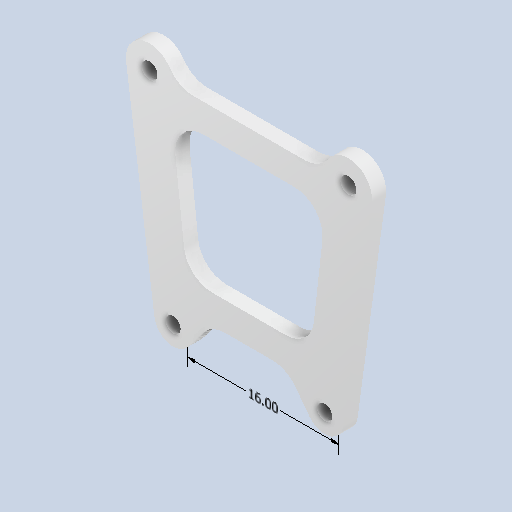
# Autodesk Inventor part: elbow
Saved by Autodesk Inventor 2024.1 (Build 281209000, 209)
## iProperties
Created: 2024-02-14
Part Number: elbow
Material: アルミニウム 6061
Document SubType Name: Modeling
Designer: hibik
Density: 2.7 g/cm^3
Appearance: アルミニウム - フラット
Author: hibik
Autodesk Inventor part; units mm, degrees
ref_plane "YZ Plane" through (0, 0, 0) normal (1, 0, 0) x (0, 1, 0)
ref_plane "XZ Plane" through (0, 0, 0) normal (0, 1, 0) x (-1, 0, 0)
ref_plane "XY Plane" through (0, 0, 0) normal (0, 0, 1) x (1, 0, 0)
sketch "スケッチ2" plane through (0, 0, 0) normal (0, 0, 1) x (1, 0, 0)
  line L0 (0, 0) -> (26, 0)
  line L1 (26, 0) -> (26, 33)
  line L2 (26, 33) -> (0, 33)
  line L3 (0, 33) -> (0, 0)
  line L4 (0, 0) -> (26, 0)
  line L5 (26, 0) -> (26, 24)
  line L6 (26, 24) -> (0, 24) construction
  line L7 (0, 24) -> (0, 0)
  circle A0 centre (13, 24) radius 13
  circle A1 centre (13, 24) radius 6.25
  line L8 (26, 0) -> (0, 0)
  line L9 (26, 24.5219) -> (26, -21)
  line L10 (26, -21) -> (0, -21)
  line L11 (0, -21) -> (0, 24)
  circle A2 centre (5, -19) radius 0.8
  circle A3 centre (21, -19) radius 0.8
  line L12 (0, 24) -> (26, 24)
  point P0 (22.3808, 33)
  point P1 (3.6192, 33)
  point P2 (0, 0)
  point P3 (26, 24)
  point P4 (0, 24)
  point P5 (6.75, 24)
  point P6 (19, 22.25)
  point P7 (19.25, 24)
  dimension "d0" = 26
  dimension "d1" = 33
  dimension "d2" = 24
  dimension "d3" = 12.5
  dimension "d14" = 26
  dimension "d17" = 1.6
  dimension "d18" = 1.6
  dimension "d19" = 2
  dimension "d20" = 2
  dimension "d21" = 5
  dimension "d22" = 5
  dimension "d23" = 13
  dimension "d25" = 45
  dimension "d26" = 0
  constraints: 26 end point, 5 parallel, 3 centre point, 3 horizontal, 3 perpendicular, 2 midpoint, 2 point on line, 1 coincident, 3 other
  measures "d0" distance of L1.end L2.end
  measures "d1" distance of L2.end L0.start
  measures "d2" distance between parallel lines of L0 L6
  measures "d3" diameter of A1
  measures "d14" distance between parallel lines of L11 L9
  measures "d17" diameter of A2
  measures "d18" diameter of A3
  measures "d19" distance from line of A2.centre L10
  measures "d20" distance from line of L10 A3.centre
  measures "d21" distance from line of L11 A2.centre
  measures "d22" distance from line of L9 A3.centre
  measures "d23" distance from line of L11 A1.centre
  measures "d25" distance between parallel lines of L10 L12
  measures "d26" distance between parallel lines of L9 L1
extrude "押し出し1" add sketch "スケッチ2" along normal blind 1.5 contours L3 A0 L1 L0 | L0 L9 L10 L11 | L12 A1 A0 | A0 L2 L12 A1 | A0 L2 L1 | L12 A1 | A1 L12
sketch "スケッチ3" plane through (0, 0, 0) normal (0, 0, -1) x (-1, 0, 0)
  circle A0 centre (-2.5, 24) radius 0.85 projected
  circle A1 centre (-23.5, 24) radius 0.85 projected
  circle A2 centre (-23.5, 3) radius 0.85 projected
  circle A3 centre (-2.5, 3) radius 0.85 projected
  circle A4 centre (-13, 24) radius 6.25 projected
  line L0 (-2.5, 24) -> (-23.5, 24)
  line L1 (-23.5, 24) -> (-23.5, 3)
  line L2 (-23.5, 3) -> (-2.5, 3)
  line L3 (-2.5, 3) -> (-2.5, 24)
  circle A5 centre (-13, 24) radius 10.25
  line L4 (-5.5, 24) -> (-20.5, 24)
  line L5 (-20.5, 24) -> (-20.5, 3)
  line L6 (-20.5, 3) -> (-5.5, 3)
  line L7 (-5.5, 3) -> (-5.5, 24)
  arc A6 (0, 24) -> (-3.6192, 33) centre (-13, 24) ccw projected
  line L8 (-26, 33) -> (-3.6192, 33) projected
  line L9 (-26, -21) -> (-26, 33) projected
  line L10 (0, -21) -> (-26, -21) projected
  line L11 (0, 24) -> (0, -21) projected
  circle A7 centre (-5, -19) radius 0.8 projected
  circle A8 centre (-21, -19) radius 0.8 projected
  line L12 (-37.149, 0) -> (-22.2321, 0)
  line L13 (-22.2321, 0) -> (-8, 0)
  circle A9 centre (-23.5, 3) radius 2.5
  circle A10 centre (-2.5, 3) radius 2.5
  line L14 (-21.5265, 4.5347) -> (-18, 0)
  line L15 (-4.4735, 4.5347) -> (-8, 0)
  line L16 (-18, 0) -> (-8, 0)
  circle A11 centre (-21, -19) radius 2
  circle A12 centre (-5, -19) radius 2
  line L17 (-26, -21) -> (-26, 33) projected
  line L18 (-19.4, -20.2) -> (-17, -17)
  line L19 (-17, -17) -> (-9, -17)
  line L20 (-9, -17) -> (-6.6, -20.2)
  line L21 (-25.977, 2.6617) -> (-22.9816, -19.2706)
  line L22 (-0.023, 2.6617) -> (-3.0184, -19.2706)
  line L23 (-23.5, 3) -> (-21, -19)
  line L24 (-2.5, 3) -> (-5, -19)
  line L25 (-23.1591, 0) -> (-2.8409, 0)
  line L26 (-21.5682, -14) -> (-4.4318, -14)
  line L27 (-21.1462, 0) -> (-19.5553, -14)
  line L28 (-4.8538, 0) -> (-6.4447, -14)
  point P0 (0, 0)
  point P1 (-5.5, 17.0134)
  point P2 (-20.5, 17.0134)
  point P3 (-13, 0)
  point P4 (-13, -21)
  point P5 (-13, -17)
  point P6 (-21, -21)
  point P7 (-5, -21)
  point P8 (-25.6135, 0)
  point P9 (-26, 0)
  point P10 (0, 3)
  point P11 (-8.0946, 33)
  point P12 (-17.9054, 33)
  point P13 (-26, 3)
  point P14 (-20.5, 3.2147)
  point P15 (-5.5, 3.2147)
  point P16 (-3.35, 3)
  point P17 (-2.5, 3.85)
  point P18 (-2.5, 5.5)
  point P19 (-23.5, 5.5)
  point P20 (-23.5, 3.85)
  point P21 (-22.65, 3)
  point P22 (-5.667, 3)
  point P23 (-20.333, 3)
  dimension "d27" = 4
  dimension "d28" = 3
  dimension "d29" = 3
  dimension "d36" = 3
  dimension "d38" = 10
  dimension "d39" = 8
  dimension "d40" = 3
  dimension "d41" = 3
  dimension "d42" = 2
  dimension "d43" = 2
  constraints: 48 end point, 13 tangent, 11 point on line, 8 point on circle, 7 coincident, 7 parallel, 5 centre point, 5 horizontal, 3 midpoint, 2 collinear, 2 perpendicular, 2 vertical alignment
  measures "d27" radial gap between concentric circles of A5 A4
  measures "d28" distance between parallel lines of L3 L7
  measures "d29" distance between parallel lines of L1 L5
  measures "d36" distance from line of L1.end L12
  measures "d38" distance of L14.end L13.end
  measures "d39" distance of L18.end L19.end
  measures "d40" distance between parallel lines of L6 L25
  measures "d41" distance between parallel lines of L19 L26
  measures "d42" distance between parallel lines of L23 L27
  measures "d43" distance between parallel lines of L24 L28
extrude "押し出し2" cut sketch "スケッチ3" against normal through all contours A0 L3 L0 A5 | A0 A5 L8 A6 L11 A10 L3 | A5 L0 A0 | A0 L0 A4 A1 A5 L8 | L3 A10 L15 L7 A5 A0 | A0 A5 L0 L3 | L0 A5 A0 | A0 A5 L7 L0 | L8 A5 | L7 A5 L5 L0 A4 | A5 A1 L1 A9 L9 L8 | L7 L15 L2 L14 L5 A5 | L3 L2 A3 | A3 L24 L3 | L11 L10 A12 L22 A10 | L0 A4 | A4 L0 | A5 L0 L1 A1 | A1 L0 A5 | L5 L14 A9 L1 A1 A5 | A5 A1 L0 L5 | L2 L24 A3 | A1 A5 L0 | L1 L0 A5 A1 | A9 L21 L12 L9 | L10 A11 L18 L19 L20 A12 | L12 L21 A11 L10 L9 | L25 L28 L26 L27 L13 | L1 L23 A2 | A2 L2 L1 | A2 L23 L2
fillet "フィレット1" radius 3 8 edges at (4.8538, 0, 0.75) (21.1462, 0, 0.75) (19.5553, -14, 0.75) (6.4447, -14, 0.75) (9, -17, 0.75) (17, -17, 0.75) (20.333, 3, 0.75) (5.667, 3, 0.75)
equation "\"d20\" = d19"
